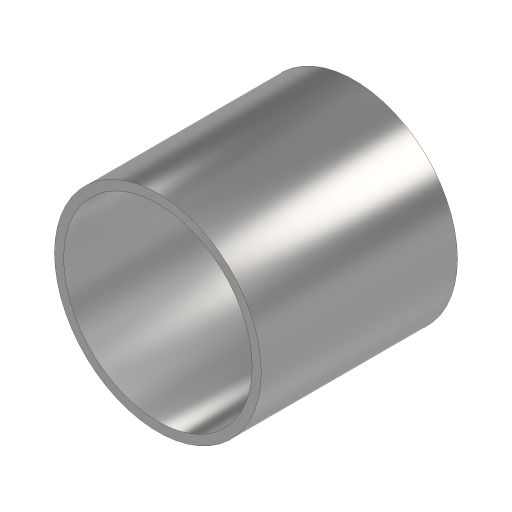
# Autodesk Inventor part: Part4
Saved by Autodesk Inventor 2024.2 (Build 282272000, 272)
## iProperties
Created: 2019-06-28
Part Number: Part4
Material: Stainless Steel
Document SubType Name: Modeling
Designer: Nakamura
Density: 8 g/cm^3
Appearance: Semi-Polished
Mass: 25.2136 g
Surface Area: 29.4485 cm^2
Volume: 3.1517 cm^3
Author: Nakamura
Autodesk Inventor part; units mm, degrees
ref_plane "YZ Plane" through (0, 0, 0) normal (1, 0, 0) x (0, 1, 0)
ref_plane "XZ Plane" through (0, 0, 0) normal (0, 1, 0) x (-1, 0, 0)
ref_plane "XY Plane" through (0, 0, 0) normal (0, 0, 1) x (1, 0, 0)
sketch "Sketch4" plane through (0, 0, 0) normal (0, 0, 1) x (1, 0, 0)
  circle A0 centre (0, 0) radius 6.25
  circle A1 centre (0, 0) radius 6.85
  dimension "d9" = 12.5
  dimension "d10" = 13.7
  constraints: 2 centre point, 2 coincident
  measures "d9" diameter of A0
  measures "d10" diameter of A1
extrude "Extrusion4" add sketch "Sketch4" along normal blind 13
body "Solid2"
